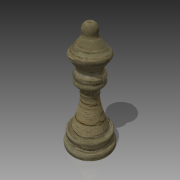
# Autodesk Inventor part: Bishop
Saved by Autodesk Inventor 2015 SP1 (Build 190203100, 203)
## iProperties
Created: 2015-06-07
Part Number: Bishop
Material: Generic
Document SubType Name: Modeling
Designer: Nathan
Density: 1 g/cm^3
Appearance: Driftwood
Author: Nathan
Autodesk Inventor part; units mm, degrees
ref_plane "YZ Plane" through (0, 0, 0) normal (1, 0, 0) x (0, 1, 0)
ref_plane "XZ Plane" through (0, 0, 0) normal (0, 1, 0) x (-1, 0, 0)
ref_plane "XY Plane" through (0, 0, 0) normal (0, 0, 1) x (1, 0, 0)
sketch "Sketch1" plane through (0, 0, 0) normal (0, 0, 1) x (1, 0, 0)
  line L0 (0, 10.7167) -> (0, 0)
  line L1 (0, 0) -> (14.846, 0)
  arc A0 (12.9584, 6.4952) -> (13.7958, 3.4613) centre (14.831, 5.3796) ccw
  line L2 (13.2402, 9.7167) -> (13.2402, 7.5188)
  line L3 (14.846, 1.7013) -> (14.846, 0)
  arc A1 (12.9584, 6.4952) -> (13.2402, 7.5188) centre (11.2402, 7.5188) ccw
  arc A2 (14.846, 1.7013) -> (13.7958, 3.4613) centre (12.846, 1.7013) ccw
  arc A3 (13.2402, 9.7167) -> (12.2402, 10.7167) centre (12.2402, 9.7167) ccw
  line L4 (0, 0) -> (0, 10.7167)
  line L5 (12.2402, 10.7167) -> (10.8438, 10.7167)
  line L6 (0, 0) -> (0, 70)
  ellipse E0 centre (0, 66.2166) end of major axis (3.9001, 66.2166) minor radius 3.7834 (3.2339, 64.1018) -> (0, 70) ccw
  line L7 (3.2339, 64.1018) -> (9.9137, 56.2495)
  line L8 (10.0197, 53.7939) -> (5.2731, 47.1249)
  spline S0 degree 4 poles (5.2731, 47.1249) (5.8904, 46.7247) (6.8309, 46.3442) (8.0883, 45.8027) (9.177, 45.2019) (9.3404, 45.1069) knots 1.249031 1.249031 1.249031 1.249031 1.249031 2 2.137857 2.137857 2.137857 2.137857 2.137857
  spline S1 degree 4 poles (5.0523, 37.298) (4.7101, 37.0822) (4.3679, 36.8472) (4.0341, 36.5946) (5.4047, 34.1495) knots 1.601121 1.601121 1.601121 1.601121 1.601121 1.745803 1.745803 1.745803 1.745803 1.745803
  line L9 (5.2731, 47.1249) -> (5.8904, 46.7247) construction
  line L10 (5.8904, 46.7247) -> (6.8309, 46.3442) construction
  arc A4 (10.0197, 53.7939) -> (9.9137, 56.2495) centre (8.3903, 54.9536) ccw
  line L11 (9.3404, 45.1069) -> (7.3485, 43.0398) construction
  line L12 (7.3485, 43.0398) -> (7.965, 42.3151) construction
  line L13 (7.965, 42.3151) -> (8.29, 41.4519) construction
  line L14 (8.29, 41.4519) -> (8.3266, 40.4438) construction
  spline S2 degree 4 poles (9.3404, 45.1069) (7.3485, 43.0398) (7.965, 42.3151) (8.29, 41.4519) (8.3266, 40.4438) (7.8656, 39.7832) (6.7164, 38.5609) (5.0523, 37.298) knots 1 1 1 1 1 2 3 4 4.951399 4.951399 4.951399 4.951399 4.951399
  line L15 (8.3266, 40.4438) -> (7.8656, 39.7832) construction
  line L16 (7.8656, 39.7832) -> (6.7164, 38.5609) construction
  line L17 (6.7164, 38.5609) -> (5.0523, 37.298) construction
  line L18 (5.0523, 37.298) -> (4.7101, 37.0822) construction
  line L19 (6.8309, 46.3442) -> (8.0883, 45.8027) construction
  line L20 (8.0883, 45.8027) -> (9.177, 45.2019) construction
  line L21 (9.177, 45.2019) -> (9.3404, 45.1069) construction
  line L22 (7.7716, 17.8018) -> (10.8438, 10.7167) construction
  spline S3 degree 4 poles (5.4047, 34.1495) (4.0772, 32.8249) (5.4727, 26.7733) (7.7716, 17.8018) (10.8438, 10.7167) knots 1.101905 1.101905 1.101905 1.101905 1.101905 2 2 2 2 2
  line L23 (5.4047, 34.1495) -> (4.0772, 32.8249) construction
  line L24 (4.0772, 32.8249) -> (5.4727, 26.7733) construction
  line L25 (5.4727, 26.7733) -> (7.7716, 17.8018) construction
  line L26 (4.7101, 37.0822) -> (4.3679, 36.8472) construction
  line L27 (4.3679, 36.8472) -> (4.0341, 36.5946) construction
  line L28 (4.0341, 36.5946) -> (5.4047, 34.1495) construction
  point P0 (14.846, 3.1999)
  point P1 (13.2402, 6.8697)
  dimension "d11" = 2
  dimension "d13" = 1
  dimension "d34" = 70
  dimension "d35" = 2
  constraints: 18 end point, 13 point on circle, 7 tangent, 5 centre point, 3 point on line, 3 vertical, 2 horizontal, 1 equal radius, 16 other
  measures "d11" radius of A1
  measures "d13" radius of A3
  measures "d34" distance of L6.end L0.end
  measures "d35" radius of A4
revolve "Revolution1" add sketch "Sketch1" angle 360 about axis through (0, 10.7167, 0) along (0, -1, 0)
fillet "Fillet3" radius 2 3 edges at (-9.3404, 45.1069, 0) (-5.4047, 34.1495, 0) (-5.2731, 47.1249, 0)
fillet "Fillet4" radius 2 1 edges at (-10.8438, 10.7167, 0)
fillet "Fillet5" radius 2 1 edges at (-3.2339, 64.1018, 0)
body "Solid1"
